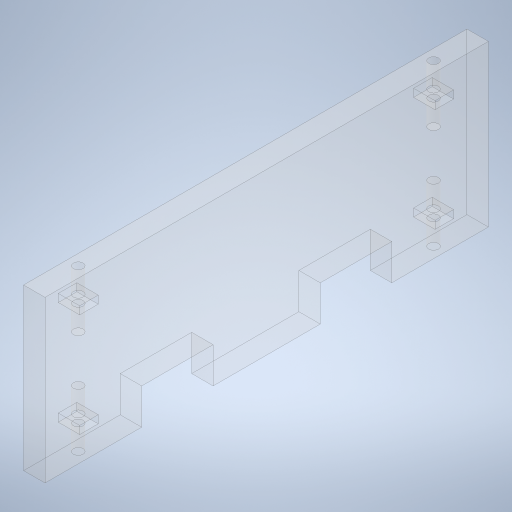
# Autodesk Inventor part: frame_head3
Saved by Autodesk Inventor 2024 (Build 280153000, 153)
## iProperties
Created: 2024-09-08
Part Number: frame_head3
Material: PMMA 플라스틱
Document SubType Name: Modeling
Designer: jmha0
Density: 1.188 g/cm^3
Appearance: 폴리카보네이트 - 선명
Author: jmha0
Autodesk Inventor part; units mm, degrees
ref_plane "YZ Plane" through (0, 0, 0) normal (1, 0, 0) x (0, 1, 0)
ref_plane "XZ Plane" through (0, 0, 0) normal (0, 1, 0) x (-1, 0, 0)
ref_plane "XY Plane" through (0, 0, 0) normal (0, 0, 1) x (1, 0, 0)
sketch "스케치1" plane through (0, 0, 0) normal (0, 1, 0) x (-1, 0, 0)
  line L0 (3.5912, -53.5318) -> (3.5912, 70.5682)
  line L1 (3.5912, -53.5318) -> (-2.4088, -53.5318)
  line L2 (-2.4088, -53.5318) -> (-2.4088, 70.5682)
  line L3 (-2.4088, 70.5682) -> (3.5912, 70.5682)
  line L4 (3.5912, 70.5682) -> (3.5912, -53.5318)
  point P0 (0, 0)
  dimension "d0" = 6
  constraints: 10 end point, 2 parallel, 1 horizontal, 1 perpendicular
  measures "d0" distance of L3.start L3.end
extrude "돌출1" add sketch "스케치1" along normal blind 45
sketch "스케치2" plane through (0, 45, 0) normal (0, 1, 0) x (1, 0, 0)
  line L0 (2.4088, -70.5682) -> (2.4088, 53.5318)
  line L1 (2.4088, -70.5682) -> (-3.5912, -70.5682)
  line L2 (-3.5912, -70.5682) -> (-3.5912, 53.5318)
  line L3 (-3.5912, 53.5318) -> (2.4088, 53.5318)
  line L4 (2.4088, 53.5318) -> (2.4088, -70.5682)
  circle A0 centre (-0.5912, -58.2682) radius 1.35
  circle A1 centre (-0.5912, 41.1925) radius 1.35
  line L5 (2.4088, -70.5682) -> (2.4088, 53.5318) projected
  line L6 (2.4088, 53.5318) -> (-3.5912, 53.5318) projected
  line L7 (-3.5912, 53.5318) -> (-3.5912, -70.5682) projected
  line L8 (-3.5912, -70.5682) -> (2.4088, -70.5682) projected
  point P0 (0, 0)
  dimension "d3" = 6
  dimension "d4" = 2.7
  dimension "d5" = 2.7
  constraints: 10 end point, 2 centre point, 2 parallel, 1 horizontal, 1 perpendicular
  measures "d3" distance of L3.start L3.end
  measures "d4" diameter of A0
  measures "d5" diameter of A1
extrude "돌출2" cut sketch "스케치2" against normal blind 16 contours A0 | A1
sketch "스케치3" plane through (2.4088, 0, 70.5682) normal (1, 0, 0) x (0, 0, -1)
  line L0 (0, 0) -> (124.1, 0) projected
  line L1 (124.1, 0) -> (124.1, 45) projected
  line L2 (0, 45) -> (124.1, 45) projected
  line L3 (0, 0) -> (0, 45) projected
  line L4 (62.05, 0) -> (77.05, 0)
  line L5 (77.05, 0) -> (47.05, 0)
  line L6 (77.05, 0) -> (97.05, 0)
  line L7 (97.05, 0) -> (97.05, 10)
  line L8 (97.05, 10) -> (77.05, 10)
  line L9 (77.05, 10) -> (77.05, 0)
  line L10 (47.05, 0) -> (27.05, 0)
  line L11 (27.05, 0) -> (27.05, 10)
  line L12 (27.05, 10) -> (47.05, 10)
  line L13 (47.05, 10) -> (47.05, 0)
  point P0 (70.5682, 0)
  dimension "d8" = 15
  dimension "d9" = 30
  dimension "d10" = 20
  dimension "d11" = 10
  dimension "d12" = 20
  dimension "d13" = 10
  constraints: 20 end point, 4 parallel, 2 horizontal, 2 perpendicular, 2 point on line, 1 midpoint
  measures "d8" distance of L4.start L4.end
  measures "d9" distance of L4.end L5.end
  measures "d10" distance of L8.end L7.end
  measures "d11" distance of L7.end L6.end
  measures "d12" distance of L11.end L12.end
  measures "d13" distance of L10.end L11.end
extrude "돌출3" cut sketch "스케치3" against normal blind 16 contours L11 L12 L13 L0 | L9 L8 L7 L0
sketch "스케치4" plane through (0, 0, 0) normal (0, -1, 0) x (1, 0, 0)
  circle A0 centre (-0.5912, 58.2682) radius 1.35 projected
  circle A1 centre (-0.5912, -41.1925) radius 1.35 projected
  point P0 (0, 0)
extrude "돌출4" cut sketch "스케치4" against normal blind 16
sketch "스케치5" plane through (2.4088, 0, -53.5318) normal (1, 0, 0) x (0, 0, -1)
  line L0 (-97.05, 0) -> (-124.1, 0) projected
  line L1 (-124.1, 0) -> (-97.05, 0) projected
  line L2 (-27.05, 0) -> (0, 0) projected
  line L3 (0, 45) -> (-124.1, 45) projected
  line L4 (-124.1, 45) -> (0, 45) projected
  line L5 (-113.15, 45) -> (-110.45, 45) projected
  line L6 (-13.6892, 45) -> (-10.9892, 45) projected
  line L7 (-124.1, 45) -> (0, 45) projected
  line L8 (0, 45) -> (-124.1, 45) projected
  line L9 (-47.05, 10) -> (-47.05, 0) projected
  line L10 (-47.05, 0) -> (-77.05, 0) projected
  line L11 (-77.05, 0) -> (-77.05, 10) projected
  line L12 (-77.05, 10) -> (-97.05, 10) projected
  line L13 (-97.05, 10) -> (-97.05, 0) projected
  line L14 (-97.05, 0) -> (-124.1, 0) projected
  line L15 (-124.1, 0) -> (-124.1, 45) projected
  line L16 (0, 45) -> (-124.1, 45) projected
  line L17 (0, 0) -> (0, 45) projected
  line L18 (0, 0) -> (-27.05, 0) projected
  line L19 (-27.05, 0) -> (-27.05, 10) projected
  line L20 (-27.05, 10) -> (-47.05, 10) projected
  line L21 (-47.05, 0) -> (-47.05, 10) projected
  line L22 (-47.05, 10) -> (-27.05, 10) projected
  line L23 (-27.05, 10) -> (-27.05, 0) projected
  line L24 (-27.05, 0) -> (0, 0) projected
  line L25 (0, 0) -> (0, 45) projected
  line L26 (-124.1, 45) -> (0, 45) projected
  line L27 (-124.1, 0) -> (-124.1, 45) projected
  line L28 (-124.1, 0) -> (-97.05, 0) projected
  line L29 (-97.05, 0) -> (-97.05, 10) projected
  line L30 (-97.05, 10) -> (-77.05, 10) projected
  line L31 (-77.05, 10) -> (-77.05, 0) projected
  line L32 (-77.05, 0) -> (-47.05, 0) projected
  line L33 (-97.05, 10) -> (-77.05, 10) projected
  line L34 (-77.05, 10) -> (-97.05, 10) projected
  line L35 (-77.05, 10) -> (-97.05, 10) projected
  line L36 (-97.05, 10) -> (-77.05, 10) projected
  line L37 (-97.05, 10) -> (-97.05, 0) projected
  line L38 (-97.05, 10) -> (-97.05, 0) projected
  line L39 (-97.05, 0) -> (-97.05, 10) projected
  line L40 (-97.05, 0) -> (-97.05, 10) projected
  line L41 (-110.45, 16) -> (-113.15, 16) projected
  line L42 (-110.45, 16) -> (-113.15, 16) projected
  line L43 (-110.45, 0) -> (-113.15, 0) projected
  line L44 (-110.45, 16) -> (-113.15, 16) projected
  line L45 (-110.45, 0) -> (-113.15, 0) projected
  line L46 (-113.15, 29) -> (-110.45, 29) projected
  line L47 (-113.15, 29) -> (-110.45, 29) projected
  line L48 (-113.15, 29) -> (-110.45, 29) projected
  line L49 (-113.15, 45) -> (-110.45, 45) projected
  line L50 (-110.45, 0) -> (-113.15, 0) projected
  line L51 (-124.1, 0) -> (-97.05, 0) projected
  line L52 (-97.05, 0) -> (-124.1, 0) projected
  line L53 (-124.1, 0) -> (-124.1, 45) projected
  line L54 (-124.1, 0) -> (-124.1, 45) projected
  line L55 (-124.1, 0) -> (-124.1, 45) projected
  line L56 (-124.1, 0) -> (-124.1, 45) projected
  line L57 (-10.9892, 16) -> (-13.6892, 16) projected
  line L58 (-10.9892, 16) -> (-13.6892, 16) projected
  line L59 (-10.9892, 0) -> (-13.6892, 0) projected
  line L60 (-10.9892, 16) -> (-13.6892, 16) projected
  line L61 (-10.9892, 0) -> (-13.6892, 0) projected
  line L62 (0, 0) -> (0, 45) projected
  line L63 (-10.9892, 0) -> (-13.6892, 0) projected
  line L64 (0, 0) -> (-27.05, 0) projected
  line L65 (-27.05, 0) -> (0, 0) projected
  line L66 (0, 0) -> (-27.05, 0) projected
  line L67 (-113.15, 45) -> (-110.45, 45) projected
  line L68 (0, 0) -> (0, 45) projected
  line L69 (-47.05, 0) -> (-47.05, 10) projected
  line L70 (-47.05, 10) -> (-47.05, 0) projected
  line L71 (-47.05, 10) -> (-47.05, 0) projected
  line L72 (-47.05, 0) -> (-47.05, 10) projected
  line L73 (-47.05, 10) -> (-27.05, 10) projected
  line L74 (-27.05, 10) -> (-47.05, 10) projected
  line L75 (-47.05, 10) -> (-27.05, 10) projected
  line L76 (-27.05, 0) -> (-27.05, 10) projected
  line L77 (-27.05, 10) -> (-27.05, 0) projected
  line L78 (-27.05, 0) -> (-27.05, 10) projected
  line L79 (-27.05, 10) -> (-27.05, 0) projected
  line L80 (-13.6892, 45) -> (-10.9892, 45) projected
  line L81 (-13.6892, 29) -> (-10.9892, 29) projected
  line L82 (-13.6892, 29) -> (-10.9892, 29) projected
  line L83 (-13.6892, 45) -> (-10.9892, 45) projected
  line L84 (0, 0) -> (0, 45) projected
  line L85 (0, 0) -> (0, 45) projected
  line L86 (-13.6892, 29) -> (-10.9892, 29) projected
  line L87 (-77.05, 10) -> (-77.05, 0) projected
  line L88 (-77.05, 0) -> (-77.05, 10) projected
  line L89 (-77.05, 10) -> (-77.05, 0) projected
  line L90 (-77.05, 0) -> (-47.05, 0) projected
  line L91 (-77.05, 0) -> (-47.05, 0) projected
  line L92 (-47.05, 0) -> (-77.05, 0) projected
  line L93 (-47.05, 0) -> (-77.05, 0) projected
  line L94 (-77.05, 0) -> (-77.05, 10) projected
  line L95 (-27.05, 10) -> (-47.05, 10) projected
  line L96 (-13.6892, 0) -> (-13.6892, 16) projected
  line L97 (-10.9892, 0) -> (-10.9892, 16) projected
  line L98 (-13.6892, 45) -> (-13.6892, 29) projected
  line L99 (-10.9892, 45) -> (-10.9892, 29) projected
  line L100 (-110.45, 45) -> (-110.45, 29) projected
  line L101 (-113.15, 45) -> (-113.15, 29) projected
  line L102 (-113.15, 0) -> (-113.15, 16) projected
  line L103 (-110.45, 0) -> (-110.45, 16) projected
  line L104 (-9.7392, 6.9) -> (-14.9392, 6.9)
  line L105 (-14.9392, 6.9) -> (-14.9392, 9.1)
  line L106 (-14.9392, 9.1) -> (-9.7392, 9.1)
  line L107 (-9.7392, 9.1) -> (-9.7392, 6.9)
  line L108 (-9.7392, 6.9) -> (-14.9392, 9.1) construction
  line L109 (-14.9392, 6.9) -> (-9.7392, 9.1) construction
  line L110 (-109.2, 9.1) -> (-114.4, 9.1)
  line L111 (-114.4, 9.1) -> (-114.4, 6.9)
  line L112 (-114.4, 6.9) -> (-109.2, 6.9)
  line L113 (-109.2, 6.9) -> (-109.2, 9.1)
  line L114 (-109.2, 9.1) -> (-114.4, 6.9) construction
  line L115 (-114.4, 9.1) -> (-109.2, 6.9) construction
  line L116 (-9.7392, 38.1) -> (-14.9392, 38.1)
  line L117 (-14.9392, 38.1) -> (-14.9392, 35.9)
  line L118 (-14.9392, 35.9) -> (-9.7392, 35.9)
  line L119 (-9.7392, 35.9) -> (-9.7392, 38.1)
  line L120 (-9.7392, 38.1) -> (-14.9392, 35.9) construction
  line L121 (-14.9392, 38.1) -> (-9.7392, 35.9) construction
  line L122 (-109.2, 35.9) -> (-114.4, 35.9)
  line L123 (-114.4, 35.9) -> (-114.4, 38.1)
  line L124 (-114.4, 38.1) -> (-109.2, 38.1)
  line L125 (-109.2, 38.1) -> (-109.2, 35.9)
  line L126 (-109.2, 35.9) -> (-114.4, 38.1) construction
  line L127 (-114.4, 35.9) -> (-109.2, 38.1) construction
  point P0 (-53.5318, 0)
  point P1 (-12.3392, 8)
  point P2 (-111.8, 8)
  point P3 (-12.3392, 37)
  point P4 (-111.8, 37)
  dimension "d18" = 5.2
  dimension "d19" = 2.2
  dimension "d20" = 5.2
  dimension "d21" = 2.2
  dimension "d22" = 5.2
  dimension "d23" = 2.2
  constraints: 48 end point, 8 midpoint, 8 parallel, 4 horizontal, 4 perpendicular, 2 point on line, 11 other
  measures "d18" distance of L105.end L106.end
  measures "d19" distance of L104.end L105.end
  measures "d20" distance of L112.end L111.end
  measures "d21" distance of L111.end L110.end
  measures "d22" distance of L118.end L117.end
  measures "d23" distance of L117.end L116.end
extrude "돌출5" cut sketch "스케치5" against normal blind 16 contours L112 L102 L110 L103 | L103 L110 L113 L112 | L112 L111 L110 L102 | L124 L100 L122 L101 | L101 L122 L123 L124 | L124 L125 L122 L100 | L116 L99 L118 L98 | L98 L118 L117 L116 | L116 L119 L118 L99 | L104 L105 L106 L96 | L96 L106 L97 L104 | L97 L106 L107 L104
